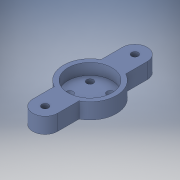
# Autodesk Inventor part: HarmonicDrive-WaveGenerator-Bottom
Saved by Autodesk Inventor 2018.3 (Build 223284000, 284)
## iProperties
Created: 2018-06-23
Part Number: HarmonicDrive-WaveGenerator-Bottom
Material: Generisch
Document SubType Name: Modeling
Designer: JochenAlt
Density: 1 g/cm^3
Appearance: Gummi - blau
Author: JochenAlt
Autodesk Inventor part; units mm, degrees
ref_plane "YZ Plane" through (0, 0, 0) normal (1, 0, 0) x (0, 1, 0)
ref_plane "XZ Plane" through (0, 0, 0) normal (0, 1, 0) x (-1, 0, 0)
ref_plane "XY Plane" through (0, 0, 0) normal (0, 0, 1) x (1, 0, 0)
sketch "Skizze1" plane through (0, 0, 0) normal (0, 0, 1) x (1, 0, 0)
  line L0 (0, -19.95) -> (0, 19.95) construction
  arc A0 (-5.5, -19.95) -> (5.5, -19.95) centre (0, -19.95) ccw
  arc A1 (5.5, 19.95) -> (-5.5, 19.95) centre (0, 19.95) ccw
  line L1 (0, 37.03) -> (0, -37.03) construction
  line L2 (-16.45, 0) -> (16.45, 0) construction
  circle A2 centre (0, 19.95) radius 1.5
  circle A3 centre (0, -19.95) radius 1.5
  circle A4 centre (0, 19.95) radius 6.5 construction
  circle A5 centre (0, -19.95) radius 6.5 construction
  line L3 (0, 26.45) -> (0, -26.45) construction
  circle A6 centre (0, 19.95) radius 2.5
  circle A7 centre (0, -19.95) radius 2.5
  circle A8 centre (0, 0) radius 9.75
  line L4 (-5.5, 19.95) -> (-5.5, 10.3833)
  line L5 (-5.5, -10.3833) -> (-5.5, -19.95)
  line L6 (5.5, -19.95) -> (5.5, -10.3833)
  line L7 (5.5, 10.3833) -> (5.5, 19.95)
  arc A9 (5.5, -10.3833) -> (5.5, 10.3833) centre (0, 0) ccw
  arc A10 (-5.5, 10.3833) -> (-5.5, -10.3833) centre (0, 0) ccw
  circle A11 centre (0, 0) radius 6.35 construction
  circle A12 centre (-4.4901, 4.4901) radius 1.5
  circle A13 centre (-4.4901, -4.4901) radius 1.5
  circle A14 centre (4.4901, -4.4901) radius 1.5
  circle A15 centre (4.4901, 4.4901) radius 1.5
  line L8 (-4.4901, 4.4901) -> (0, 0) construction
  dimension "d4" = 13
  dimension "d31" = 12.7
  dimension "d1" = 3
  dimension "d5" = 52.9
  dimension "d19" = 1
  dimension "d26" = 19.5
  dimension "d28" = 2
  dimension "d32" = 3
  dimension "d35" = 360
  dimension "d37" = 45
  dimension "d38" = 3
  constraints: 16 end point, 13 centre point, 9 coincident, 8 point on circle, 8 tangent, 4 parallel, 3 equal radius, 2 midpoint, 2 point on line, 2 vertical alignment, 1 vertical, 16 other
  measures "d1" diameter of A2
  measures "d5" distance of L3.start L3.end
  measures "d19" radial gap between concentric circles of A2 A6
  measures "d26" diameter of A8
  measures "d28" radial gap between concentric circles of A8 A9
  measures "d32" diameter of A12
  measures "d37" angle of L0 L8
  measures "d38" radial gap between concentric circles of A1 A6
extrude "Extrusion1" add sketch "Skizze1" against normal blind 7 contours L5 A10 L4 A1 L7 A9 L6 A0 | A6 | A7
extrude "Extrusion4" add sketch "Skizze1" against normal blind 0.5 from surface at -7 contours A6 | A7
extrude "Extrusion6" add sketch "Skizze1" along normal blind 2 from surface at -7 contours A8
